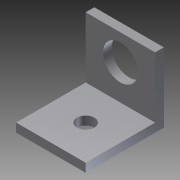
# Autodesk Inventor part: Piston Mounting Bracket
Saved by Autodesk Inventor 2012 (Build 160160000, 160)
## iProperties
Created: 2013-01-17
Part Number: Piston Mounting Bracket
Material: Default
Document SubType Name: Modeling
Designer: William
Density: 1 g/cm^3
Mass: 3.59402 g
Surface Area: 29.3783 cm^2
Volume: 3.59402 cm^3
Author: William
Autodesk Inventor part; units mm, degrees
ref_plane "YZ Plane" through (0, 0, 0) normal (1, 0, 0) x (0, 1, 0)
ref_plane "XZ Plane" through (0, 0, 0) normal (0, 1, 0) x (-1, 0, 0)
ref_plane "XY Plane" through (0, 0, 0) normal (0, 0, 1) x (1, 0, 0)
sketch "Sketch1" plane through (0, 0, 0) normal (0, 0, 1) x (1, 0, 0)
  line L0 (9.1118, -9.9057) -> (-16.2882, -9.9057)
  line L1 (-16.2882, -9.9057) -> (-16.2882, 15.4943)
  line L2 (-16.2882, 15.4943) -> (9.1118, 15.4943)
  line L3 (9.1118, 15.4943) -> (9.1118, -9.9057)
  circle A0 centre (-3.5882, 5.9693) radius 6.35
  point P0 (0, 0)
  dimension "d0" = 25.4
  dimension "d1" = 25.4
  dimension "d2" = 12.7
  dimension "d16" = 9.525
  constraints: 8 end point, 2 parallel, 1 centre point, 1 horizontal, 1 perpendicular
  measures "d0" distance of L1.end L2.end
  measures "d1" distance of L0.end L1.end
  measures "d2" diameter of A0
  measures "d16" distance from line of L2 A0.centre
extrude "Extrusion1" add sketch "Sketch1" along normal blind 3.175
sketch "Sketch2" plane through (0, 0, 3.175) normal (0, 0, 1) x (1, 0, 0)
  line L0 (9.1118, 15.4943) -> (9.1118, -9.9057) projected
  line L1 (-16.2882, -9.9057) -> (9.1118, -9.9057)
  line L2 (9.1118, -9.9057) -> (9.1118, -6.7307)
  line L3 (9.1118, -6.7307) -> (-16.2882, -6.7307)
  line L4 (-16.2882, -6.7307) -> (-16.2882, -9.9057)
  point P0 (0, 0)
  dimension "d5" = 3.175
  constraints: 8 end point, 2 parallel, 1 horizontal, 1 perpendicular, 1 point on line
  measures "d5" distance of L2.end L1.end
extrude "Extrusion2" add sketch "Sketch2" along normal blind 25.4
sketch "Sketch3" plane through (-16.2882, -6.7307, 3.175) normal (0, 1, 0) x (1, 0, 0)
  line L0 (0, -25.4) -> (25.4, -25.4) projected
  line L1 (25.4, 0) -> (25.4, -25.4) projected
  circle A0 centre (12.7, -12.7) radius 3.175
  point P0 (16.2882, 3.175)
  dimension "d9" = 6.35
  dimension "d11" = 12.7
  dimension "d13" = 12.7
  constraints: 1 centre point
  measures "d9" diameter of A0
  measures "d11" distance from line of L1 A0.centre
  measures "d13" distance from line of L0 A0.centre
extrude "Extrusion3" cut sketch "Sketch3" against normal blind 25.4
body "Solid1"
